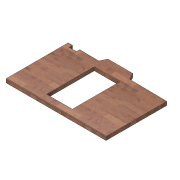
# Autodesk Inventor part: stoveCountertop
Saved by Autodesk Inventor 2018 (Build 220112000, 112)
## iProperties
Created: 2017-12-11
Part Number: stoveCountertop
Material: Wood (Maple)
Document SubType Name: Modeling
Designer: sawaiz
Density: 0.67 g/cm^3
Appearance: Wild Cherry - Whisky
Author: sawaiz
Autodesk Inventor part; units mm, degrees
ref_plane "YZ Plane" through (0, 0, 0) normal (1, 0, 0) x (0, 1, 0)
ref_plane "XZ Plane" through (0, 0, 0) normal (0, 1, 0) x (-1, 0, 0)
ref_plane "XY Plane" through (0, 0, 0) normal (0, 0, 1) x (1, 0, 0)
sketch "Sketch1" plane through (0, 0, 0) normal (0, 1, 0) x (-1, 0, 0)
  line L0 (522.5, -324.796) -> (-522.5, -310.204)
  line L1 (-522.5, -310.204) -> (-522.5, 324.796)
  line L2 (-522.5, 324.796) -> (522.5, 324.796)
  line L3 (522.5, 324.796) -> (522.5, -324.796)
  line L4 (522.5, 324.796) -> (-522.5, -310.204) construction
  line L5 (522.5, -324.796) -> (-522.5, 324.796) construction
  point P0 (0, 0)
  point P1 (0, 0)
  dimension "d2" = 635
  dimension "d26" = 1045
  dimension "d27" = 90.8
  constraints: 12 end point, 1 coincident, 1 midpoint, 1 parallel, 1 vertical, 1 other
  measures "d2" distance of L0.end L1.end
  measures "d26" distance between parallel lines of L3 L1
  measures "d27" angle of L0 L1
extrude "Extrusion1" add sketch "Sketch1" along normal blind 38
chamfer "Chamfer1" distance 5 angle 45 1 edges at (0, 38, 324.796)
sketch "Sketch3" plane through (0, 38, 0) normal (0, 1, 0) x (1, 0, 0)
  line L0 (522.5, -319.796) -> (-522.5, -319.796) projected
  line L1 (522.5, -319.796) -> (522.5, 310.204) projected
  line L2 (522.5, 310.204) -> (-522.5, 324.796) projected
  line L3 (-522.5, 324.796) -> (-522.5, -319.796) projected
  line L4 (127.786, 315.7157) -> (91.6238, 385.204)
  line L5 (91.6238, 385.204) -> (-166.9743, 385.204)
  line L6 (-166.9743, 385.204) -> (-198.1178, 320.2664)
  line L7 (-522.5, 324.796) -> (522.5, 310.204) projected
  line L8 (-522.5, -324.796) -> (522.5, -324.796) projected
  point P0 (0, 0)
  dimension "d28" = 710
  constraints: 6 end point, 2 point on line, 1 horizontal, 1 parallel
  measures "d28" distance between parallel lines of L8 L5
extrude "Extrusion3" add sketch "Sketch3" against normal up to surface (38 mm away) contours L2 L6 L5 L4
sketch "Sketch4" plane through (0, 38, 0) normal (0, 1, 0) x (1, 0, 0)
  line L0 (-170.1407, -254.5401) -> (99.8593, -254.5401)
  line L1 (99.8593, -254.5401) -> (99.8593, 245.4599)
  line L2 (99.8593, 245.4599) -> (-170.1407, 245.4599)
  line L3 (-170.1407, 245.4599) -> (-170.1407, -254.5401)
  line L4 (-170.1407, -254.5401) -> (99.8593, 245.4599) construction
  line L5 (99.8593, -254.5401) -> (-170.1407, 245.4599) construction
  line L6 (-198.0288, 315.7157) -> (127.786, 315.7157) construction
  line L7 (-170.1407, 245.4599) -> (-170.1407, 315.7157) construction
  line L8 (-170.1407, -254.5401) -> (-170.1407, -324.796) construction
  line L9 (522.5, -324.796) -> (-522.5, -324.796) projected
  point P0 (0, 0)
  point P1 (-35.1407, -4.5401)
  dimension "d21" = 270
  dimension "d22" = 500
  dimension "d25" = 70.2558
  constraints: 18 end point, 2 horizontal, 2 midpoint, 2 parallel, 2 perpendicular, 2 point on line, 1 collinear, 1 vertical
  measures "d21" distance of L2.end L1.end
  measures "d22" distance of L1.end L0.end
  measures "d25" distance of L2.end L7.end
extrude "Extrusion4" cut sketch "Sketch4" against normal through all
sketch "Sketch5" plane through (0, 38, 0) normal (0, 1, 0) x (1, 0, 0)
  line L0 (-400.1623, 288.5697) -> (-476.8678, 288.5697)
  line L1 (-476.8678, 288.5697) -> (-476.8678, 332.4674)
  line L2 (-476.8678, 332.4674) -> (-400.1623, 332.4674)
  line L3 (-400.1623, 332.4674) -> (-400.1623, 288.5697)
  point P0 (0, 0)
  constraints: 8 end point, 2 parallel, 1 horizontal, 1 perpendicular
extrude "Extrusion5" cut sketch "Sketch5" against normal through all
equation "\"d2\" = counterDepth"
equation "\"lumberWidth\" = 58"
equation "\"lumberDepth\" = 108"
equation "\"counterThickness\" = 38"
equation "\"counterHeight\" = 858"
equation "\"counterDepth\" = 635"
body "Solid1"
